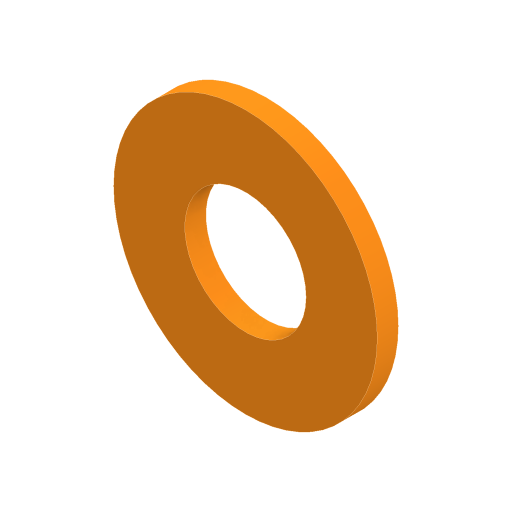
# Autodesk Inventor part: washer
Saved by Autodesk Inventor 2023 (Build 270158000, 158)
## iProperties
Created: 2023-09-14
Part Number: washer
Material: Generic
Document SubType Name: Modeling
Designer: Aditya
Density: 1 g/cm^3
Appearance: Orange
Author: Aditya
Autodesk Inventor part; units mm, degrees
ref_plane "YZ Plane" through (0, 0, 0) normal (1, 0, 0) x (0, 1, 0)
ref_plane "XZ Plane" through (0, 0, 0) normal (0, 1, 0) x (-1, 0, 0)
ref_plane "XY Plane" through (0, 0, 0) normal (0, 0, 1) x (1, 0, 0)
sketch "Sketch1" plane through (0, 0, 0) normal (0, 0, 1) x (1, 0, 0)
  circle A0 centre (0, 0) radius 1.15
  circle A1 centre (0, 0) radius 2.5
  circle A2 centre (0, 0) radius 1 construction
  dimension "shaftDia" = 2
  dimension "d1" = 0.15
  dimension "d2" = 5
  constraints: 3 centre point, 3 coincident
  measures "shaftDia" diameter of A2
  measures "d1" radial gap between concentric circles of A0 A2
  measures "d2" diameter of A1
extrude "Extrusion2" add sketch "Sketch1" along normal mid plane 0.4
equation "\"d5\" = 2 * layer"
equation "\"layer\" = 0.2"
body "Solid2"
